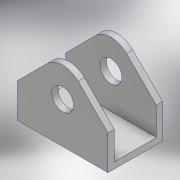
# Autodesk Inventor part: clip
Saved by Autodesk Inventor 2018.2 (Build 222227000, 227)
## iProperties
Created: 2017-12-11
Part Number: clip
Material: アルミニウム 6061
Document SubType Name: Modeling
Designer: kuwano
Density: 2.7 g/cm^3
Appearance: アルミニウム - フラット
Author: kuwano
Autodesk Inventor part; units mm, degrees
ref_plane "YZ Plane" through (0, 0, 0) normal (1, 0, 0) x (0, 1, 0)
ref_plane "XZ Plane" through (0, 0, 0) normal (0, 1, 0) x (-1, 0, 0)
ref_plane "XY Plane" through (0, 0, 0) normal (0, 0, 1) x (1, 0, 0)
sketch "スケッチ1" plane through (0, 0, 0) normal (0, 1, 0) x (-1, 0, 0)
  line L0 (0, 16.5925) -> (16.5925, 0)
  line L1 (0, 16.5925) -> (-16.5925, 0)
  line L2 (-16.5925, 0) -> (-16.5925, -12.5795)
  line L3 (-16.5925, -12.5795) -> (16.5925, -12.5795)
  line L4 (16.5925, -12.5795) -> (16.5925, 0)
  line L5 (0, -18.4139) -> (0, 22.427) projected
  line L6 (23.2296, 0) -> (-23.2296, 0) projected
  point P0 (0, 0)
  point P1 (0, -12.5795)
  dimension "d0" = 90
  constraints: 10 end point, 4 point on line, 2 perpendicular, 1 midpoint, 1 vertical
  measures "d0" angle of L1 L0
extrude "押し出し1" add sketch "スケッチ1" along normal mid plane 20
shell "シェル1" thickness 2.3 removed faces 4 at (-11.0617, 3.3333, 5.5308) at (-16.5925, 3.3333, -8.3863) at (5.5308, 3.3333, 11.0617) at (16.5925, 3.3333, -4.1932)
sketch "スケッチ3" plane through (16.5925, 10, -12.5795) normal (0, 0, -1) x (-1, 0, 0)
  circle A0 centre (16.5925, -10) radius 4
  dimension "d9" = 8
  constraints: 1 centre point, 1 coincident
  measures "d9" diameter of A0
extrude "押し出し3" cut sketch "スケッチ3" against normal through all
sketch "スケッチ4" plane through (0, 10, 0) normal (0, 1, 0) x (1, 0, 0)
  circle A0 centre (0, -2.4504) radius 4
  line L0 (0, -16.5925) -> (16.5925, 0) projected
  line L1 (-16.5925, 0) -> (0, -16.5925) projected
  point P0 (0, 0)
  dimension "d12" = 10
  dimension "d13" = 10
  dimension "d14" = 8
  constraints: 1 centre point
  measures "d12" distance from line of L0 A0.centre
  measures "d13" distance from line of L1 A0.centre
  measures "d14" diameter of A0
extrude "押し出し4" cut sketch "スケッチ4" against normal through all
fillet "フィレット1" radius 8 2 edges at (0, 8.85, 16.5925) (0, -8.85, 16.5925)
